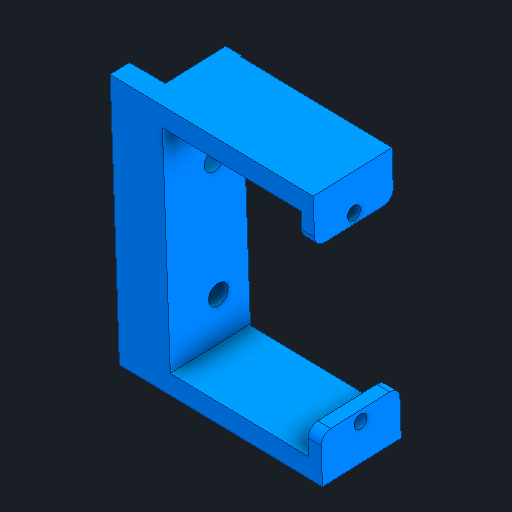
# Autodesk Inventor part: servo_mount
Saved by Autodesk Inventor 2024 (Build 280153000, 153)
## iProperties
Created: 2022-03-29
Part Number: servo_mount
Material: Generic
Document SubType Name: Modeling
Designer: kardo
Density: 1 g/cm^3
Appearance: Blue Plastic
Mass: 3.98751 g
Surface Area: 36.8709 cm^2
Volume: 3.98751 cm^3
Author: kardo
Autodesk Inventor part; units mm, degrees
ref_plane "YZ Plane" through (0, 0, 0) normal (1, 0, 0) x (0, 1, 0)
ref_plane "XZ Plane" through (0, 0, 0) normal (0, 1, 0) x (-1, 0, 0)
ref_plane "XY Plane" through (0, 0, 0) normal (0, 0, 1) x (1, 0, 0)
derived "stencil_frame.ipt"
sketch "sk_servo_mount" plane through (-54.6, 0, 0) normal (1, 0, 0) x (0, 1, 0)
  line L0 (-241.5001, 19.2432) -> (11.22, 28.376) construction
  line L1 (-345, 3089.1136) -> (-345, -1866.0023) construction
  line L2 (0, 3089.1136) -> (0, -1866.0023) construction
  line L3 (-208.8702, 20.4224) -> (-209.0941, 26.6183) construction
  line L4 (-209.0941, 26.6183) -> (-191.1059, 27.2684) construction
  line L5 (-191.1059, 27.2684) -> (-190.882, 21.0724) construction
  point P0 (0, 0)
  point P1 (-200.1, 26.9434)
ref_plane "plane_cowl_left" through (-54.6, 0, 0) normal (1, 0, 0) x (0, 1, 0)
derived "parameters_frame.ipt"
derived "parameters_powertrain.ipt"
derived "parameters_hardware.ipt"
ref_plane "plane_inner_stringer" through (-54.6, -241.5001, 19.2432) normal (1, 0, 0) x (0, 0.9993477, 0.0361144)
ref_plane "plane_fastening" through (-28.6, -241.5001, 19.2432) normal (1, 0, 0) x (0, 0.9993477, 0.0361144)
ref_plane "plane_servo_rod_joint" through (-14.6, -241.5001, 19.2432) normal (1, 0, 0) x (0, 0.9993477, 0.0361144)
ref_plane "plane_column_bottom" through (-52.1, -241.5001, 19.2432) normal (1, 0, 0) x (0, 0.9993477, 0.0361144)
ref_plane "plane_outer_plate" through (-58.1, -241.5001, 19.2432) normal (1, 0, 0) x (0, 0.9993477, 0.0361144)
ref_plane "plane_column_top" through (-30.6, -241.5001, 19.2432) normal (1, 0, 0) x (0, 0.9993477, 0.0361144)
sketch "sk_fastening" plane through (-28.6, -241.5001, 19.2432) normal (1, 0, 0) x (0, 0.9993477, 0.0361144)
  line L0 (32.6512, 6.2) -> (50.6512, 6.2) construction
  line L1 (41.6512, 6.2) -> (41.6512, 106.2) construction
  line L2 (41.6512, 106.2) -> (141.6512, 106.2) construction
  line L3 (141.6512, 106.2) -> (141.6512, 22.2) construction
  line L4 (141.6512, 22.2) -> (47.6512, 22.2) construction
  line L5 (47.6512, 22.2) -> (47.6512, 8.2) construction
  line L6 (47.6512, 8.2) -> (42.6512, 8.2) construction
  line L7 (26.1512, 14.2) -> (26.1512, 2.2)
  line L8 (26.1512, 2.2) -> (30.1512, 2.2)
  line L9 (30.1512, 2.2) -> (30.1512, 14.2)
  line L10 (30.1512, 14.2) -> (26.1512, 14.2)
  line L11 (55.1512, 14.2) -> (55.1512, 2.2)
  line L12 (55.1512, 2.2) -> (59.1512, 2.2)
  line L13 (59.1512, 2.2) -> (59.1512, 14.2)
  line L14 (59.1512, 14.2) -> (55.1512, 14.2)
  line L15 (30.1512, 14.2) -> (55.1512, 14.2) construction
  line L16 (55.1512, 2.2) -> (30.1512, 2.2) construction
  line L17 (42.6512, 2.2) -> (42.6512, 14.2) construction
  line L18 (26.1512, 14.2) -> (23.1512, 14.2)
  line L19 (23.1512, 14.2) -> (23.1512, 2.2)
  line L20 (23.1512, 2.2) -> (26.1512, 2.2)
  line L21 (59.1512, 14.2) -> (62.1512, 14.2)
  line L22 (62.1512, 14.2) -> (62.1512, 2.2)
  line L23 (62.1512, 2.2) -> (59.1512, 2.2)
  line L24 (28.6512, 8.2) -> (30.1512, 8.2) construction
  line L25 (55.1512, 8.2) -> (56.6512, 8.2) construction
  point P0 (240.6476, -27.9523)
  dimension "d46" = 100
  dimension "d47" = 84
  dimension "d49" = 100
  dimension "d50" = 94
  dimension "d52" = 14
  dimension "d53" = 5
  dimension "d54" = 25
  dimension "d55" = 33
  dimension "d56" = 3
  dimension "d57" = 3
  dimension "d58" = 12
  dimension "d59" = 28
  constraints: 50 end point, 8 collinear, 8 perpendicular, 7 parallel, 5 midpoint, 2 point on line, 1 coincident, 1 other
  measures "d46" distance of L1.end L2.end
  measures "d47" distance of L2.end L3.end
  measures "d49" distance of L1.start L1.end
  measures "d50" distance of L3.end L4.end
  measures "d52" distance of L4.end L5.end
  measures "d53" distance of L6.end L5.end
  measures "d54" distance between parallel lines of L11 L9
  measures "d55" distance between parallel lines of L13 L7
  measures "d56" distance of L7.start L18.end
  measures "d57" distance of L13.end L21.end
  measures "d58" distance of L21.end L22.end
  measures "d59" distance of L25.end L24.start
sketch "sk_base" plane through (-54.6, -241.5001, 19.2432) normal (1, 0, 0) x (0, 0.9993477, 0.0361144)
  line L0 (26.1512, 14.2) -> (23.1512, 14.2) construction
  line L1 (23.1512, 14.2) -> (23.1512, 2.2) construction
  line L2 (23.1512, 2.2) -> (26.1512, 2.2) construction
  line L3 (62.1512, 2.2) -> (59.1512, 2.2) construction
  line L4 (62.1512, 14.2) -> (62.1512, 2.2) construction
  line L5 (59.1512, 14.2) -> (62.1512, 14.2) construction
  line L6 (32.6512, 6.2) -> (50.6512, 6.2) construction
  line L7 (0, 0) -> (252.8851, 0) construction
  line L8 (23.1512, 1.5) -> (62.1512, 1.5)
  line L9 (62.1512, 1.5) -> (62.1512, 13.7)
  line L10 (62.1512, 13.7) -> (23.1512, 13.7)
  line L11 (23.1512, 13.7) -> (23.1512, 1.5)
  line L12 (32.6512, 6.2) -> (23.1512, 6.2) construction
  line L13 (32.6512, 6.2) -> (32.6512, 13.7) construction
  line L14 (50.6512, 6.2) -> (62.1512, 6.2) construction
  line L15 (50.6512, 6.2) -> (50.6512, 13.7) construction
  point P0 (240.6476, -27.9523)
  point P1 (42.6512, 8.2)
  point P2 (41.6512, 6.2)
  dimension "d60" = 20.5
  dimension "d61" = 18.5
  dimension "d62" = 18
  dimension "d64" = 1.5
  dimension "d65" = 7.5
  dimension "d66" = 18.5
  dimension "d67" = 20.5
  constraints: 16 end point, 6 perpendicular, 4 point on line, 2 parallel
  measures "d60" distance from line of L4 point (41.651, 6.2)
  measures "d61" distance from line of L1 point (41.651, 6.2)
  measures "d62" distance of L6.start L6.end
  measures "d64" distance between parallel lines of L7 L8
  measures "d65" distance of L12.start L13.end
  measures "d66" distance from line of point (41.651, 6.2) L11
  measures "d67" distance from line of point (41.651, 6.2) L9
sketch3d "sweep_axis"
sketch "sk_hex_holes" plane through (-58.1, -241.5001, 19.2432) normal (1, 0, 0) x (0, 0.9993477, 0.0361144)
  line L0 (34.2389, 8.95) -> (35.8266, 6.2)
  line L1 (35.8266, 6.2) -> (34.2389, 3.45)
  line L2 (34.2389, 3.45) -> (31.0635, 3.45)
  line L3 (31.0635, 3.45) -> (29.4758, 6.2)
  line L4 (29.4758, 6.2) -> (31.0635, 8.95)
  line L5 (31.0635, 8.95) -> (34.2389, 8.95)
  line L6 (52.2389, 8.95) -> (53.8266, 6.2)
  line L7 (53.8266, 6.2) -> (52.2389, 3.45)
  line L8 (52.2389, 3.45) -> (49.0635, 3.45)
  line L9 (49.0635, 3.45) -> (47.4758, 6.2)
  line L10 (47.4758, 6.2) -> (49.0635, 8.95)
  line L11 (49.0635, 8.95) -> (52.2389, 8.95)
  line L12 (32.6512, 6.2) -> (50.6512, 6.2) construction
  line L13 (31.0635, 3.45) -> (31.0635, -13.05)
  line L14 (31.0635, -13.05) -> (34.2389, -13.05)
  line L15 (34.2389, -13.05) -> (34.2389, 3.45)
  line L16 (49.0635, 3.45) -> (49.0635, -13.05)
  line L17 (49.0635, -13.05) -> (52.2389, -13.05)
  line L18 (52.2389, -13.05) -> (52.2389, 3.45)
  point P0 (240.6476, -27.9523)
  dimension "d102" = 5.5
  dimension "d120" = 16.5
  constraints: 38 end point, 4 perpendicular, 2 coincident, 2 collinear, 2 point on line, 1 parallel, 26 other
  measures "d102" distance between parallel lines of L2 L5
  measures "d120" distance of L2.end L13.end
sketch "sk_bridge" plane through (-54.6, -241.5001, 19.2432) normal (1, 0, 0) x (0, 0.9993477, 0.0361144)
  line L0 (62.1512, 13.7) -> (23.1512, 13.7) projected
  line L1 (23.1512, 13.7) -> (23.1512, 1.5) projected
  line L2 (62.1512, 1.5) -> (62.1512, 13.7) projected
  line L3 (23.1512, 10.7) -> (62.1512, 10.7)
  point P0 (240.6476, -27.9523)
  dimension "d70" = 3
  constraints: 2 end point, 2 point on line, 1 parallel
  measures "d70" distance between parallel lines of L0 L3
sketch "sk_backplate" plane through (-58.1, -241.5001, 19.2432) normal (1, 0, 0) x (0, 0.9993477, 0.0361144)
  line L0 (52.2389, 3.45) -> (49.0635, 3.45) projected
  line L1 (34.2389, 3.45) -> (31.0635, 3.45) projected
  line L2 (62.1512, 13.6327) -> (62.1512, 10.7)
  line L3 (55.4143, 3.45) -> (52.2389, 3.45)
  line L4 (49.0635, 3.45) -> (34.2389, 3.45)
  line L5 (31.0635, 3.45) -> (27.888, 3.45)
  line L6 (23.1512, 13.6327) -> (23.1512, 10.7)
  line L7 (31.0635, 3.45) -> (29.4758, 6.2) construction
  line L8 (23.1512, 10.7) -> (62.1512, 10.7) construction
  line L9 (53.8266, 6.2) -> (52.2389, 3.45) construction
  line L10 (27.888, 3.45) -> (26.3003, 6.2)
  line L11 (26.3003, 6.2) -> (23.1512, 10.7)
  line L12 (62.1512, 10.7) -> (57.002, 6.2)
  line L13 (57.002, 6.2) -> (55.4143, 3.45)
  line L14 (62.1512, 13.6327) -> (23.1512, 13.6327)
  point P0 (240.6476, -27.9523)
  constraints: 20 end point, 4 equal length, 3 parallel, 2 collinear, 1 coincident, 1 perpendicular
sketch3d "sweep_axis_fasterning"
  line L0 (-28.6, -179.9023, 35.6785) -> (-52.1, -179.886, 35.2269)
sweep "sweep_fastening" add profiles "sk_fastening" path "sweep_axis_fasterning" contours L7 L20 L19 L18 | L21 L22 L23 L13
sketch3d "sweep_axis_fastening_plate"
  line L0 (-28.6, -186.8977, 35.4257) -> (-30.6, -186.8963, 35.3873)
sweep "sweep_fastening_plates" add profiles "sk_fastening" path "sweep_axis_fastening_plate" contours L10 L9 L8 L7 | L14 L13 L12 L11
sketch3d "sweep_axis_front_plate"
  line L0 (-54.6, -179.8842, 35.1788) -> (-52.1, -179.886, 35.2269)
sweep "sweep_front_plate" add profiles "sk_base" path "sweep_axis_front_plate"
sketch3d "sweep_axis_bridge"
  line L0 (-54.6, -179.8842, 35.1788) -> (-58.1, -179.8818, 35.1116)
sweep "sweep_bridge" add profiles "sk_bridge" path "sweep_axis_bridge"
sketch3d "sweep_axis_backplate"
  line L0 (-58.1, -179.8818, 35.1116) -> (-60.1, -179.8804, 35.0731)
  dimension "d117" = -2
sweep "sweep_back_plate" add profiles "sk_backplate" path "sweep_axis_backplate"
extrude "_hex_holes" cut sketch "sk_hex_holes" against normal through all
hole "_fastening_holes" at (-28.6, -185.182, 29.4838) at (-28.6, -213.1637, 28.4726) direction (-1, 0, 0) diameter 2 depth 2 tip angle 118
hole "_base_holes" at (-54.6, -191.1059, 27.2684) at (-54.6, -209.0941, 26.6183) direction (1, 0, 0) diameter 3 depth 2.5 tip angle 118
fillet "fillet_1" radius 1.5 4 edges at (-29.6, -186.4637, 23.4143) (-29.6, -186.897, 35.4065) (-29.6, -211.8807, 34.5036) (-29.6, -211.4473, 22.5114)
fillet "fillet_2" radius 1.5 4 edges at (-59.1, -186.2458, 24.673) (-59.1, -184.7585, 27.4785) (-59.1, -213.7542, 23.6789) (-59.1, -215.4401, 26.3698)
equation "\"d52\" = servo_arm_length"
equation "\"d53\" = servo_axis_location"
equation "\"d55\" = servo_length_fastening"
equation "\"d58\" = servo_width"
equation "\"d59\" = servo_fastening_distance"
equation "\"d44\" = servo_height_fastening - servo_height_joint"
equation "\"servo_arm_length\" = 14"
equation "\"servo_axis_location\" = 5"
equation "\"servo_length_fastening\" = 33"
equation "\"servo_width\" = 12"
equation "\"servo_fastening_distance\" = 28"
equation "\"servo_height_fastening\" = 20"
equation "\"servo_height_joint\" = 34"
body "Solid2"
body "Solid3"
